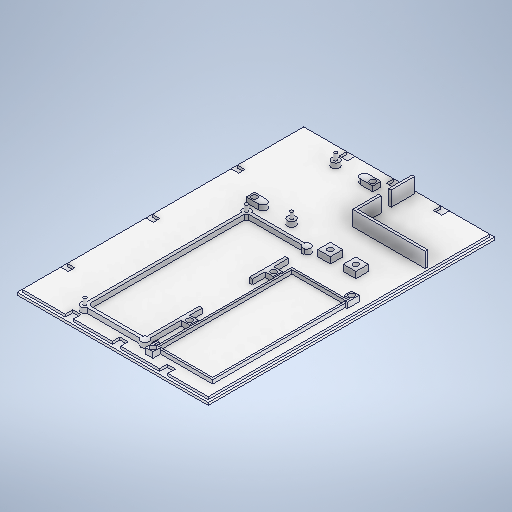
# Autodesk Inventor part: baseplate
Saved by Autodesk Inventor 2025 (Build 290162000, 162)
## iProperties
Created: 2025-05-12
Part Number: baseplate
Material: Generic
Document SubType Name: Modeling
Designer: ethan
Density: 1 g/cm^3
Appearance: PTFE
Author: ethan
Autodesk Inventor part; units mm, degrees
ref_plane "YZ Plane" through (0, 0, 0) normal (1, 0, 0) x (0, 1, 0)
ref_plane "XZ Plane" through (0, 0, 0) normal (0, 1, 0) x (-1, 0, 0)
sketch "Sketch1" plane through (0, 0, 0) normal (0, 1, 0) x (-1, 0, 0)
  line L0 (0, 0) -> (152.4, 0)
  line L1 (152.4, 0) -> (152.4, -228.6)
  line L2 (152.4, -228.6) -> (0, -228.6)
  line L3 (0, -228.6) -> (0, 0)
  dimension "d0" = 152.4
  dimension "d1" = 228.6
  constraints: 8 end point, 2 parallel, 1 horizontal, 1 perpendicular
  measures "d0" distance of L1.end L2.end
  measures "d1" distance of L0.end L1.end
extrude "BasePlate" add sketch "Sketch1" along normal blind 4
sketch "Template" plane through (0, 4, 0) normal (0, 1, 0) x (1, 0, 0)
  line L0 (0, 228.6) -> (-152.4, 228.6) construction
  line L1 (-152.4, 228.6) -> (-152.4, 0) construction
  line L2 (-152.4, 0) -> (0, 0) construction
  line L3 (0, 0) -> (0, 228.6) construction
  line L4 (-146.4, 6) -> (-146.4, 222.6) construction
  line L5 (-146.4, 222.6) -> (-6, 222.6) construction
  line L6 (-6, 222.6) -> (-6, 6) construction
  line L7 (-6, 6) -> (-146.4, 6) construction
  line L8 (-110.934, 6) -> (-110.934, 12.5) construction
  circle A0 centre (-110.934, 12.5) radius 1.25 construction
  line L9 (-110.934, 12.5) -> (-62.934, 12.5) construction
  line L10 (-62.934, 12.5) -> (-62.934, 141.5) construction
  line L11 (-62.934, 141.5) -> (-110.934, 141.5) construction
  line L12 (-110.934, 141.5) -> (-110.934, 12.5) construction
  circle A1 centre (-62.934, 12.5) radius 1.25 construction
  circle A2 centre (-110.934, 141.5) radius 1.25 construction
  circle A3 centre (-62.934, 141.5) radius 1.25 construction
  line L13 (-62.934, 12.5) -> (-6, 12.5) construction
  line L14 (-6, 12.5) -> (-9, 12.5) construction
  line L15 (-9, 12.5) -> (-55, 12.5) construction
  line L16 (-55, 12.5) -> (-55, 121.75) construction
  line L17 (-55, 121.75) -> (-9, 121.75) construction
  line L18 (-9, 121.75) -> (-9, 12.5) construction
  line L19 (-6, 222.6) -> (-63.92, 222.6) construction
  line L20 (-63.92, 222.6) -> (-63.92, 175.1) construction
  line L21 (-63.92, 175.1) -> (-6, 175.1) construction
  line L22 (-6, 175.1) -> (-6, 222.6) construction
  line L23 (-63.92, 222.6) -> (-65.92, 222.6) construction
  line L24 (-65.92, 222.6) -> (-65.92, 175.1) construction
  line L25 (-65.92, 175.1) -> (-63.92, 175.1) construction
  line L26 (-63.92, 175.1) -> (-63.92, 222.6) construction
  line L27 (-63.92, 175.1) -> (-6, 175.1) construction
  line L28 (-6, 175.1) -> (-6, 173.1) construction
  line L29 (-6, 173.1) -> (-63.92, 173.1) construction
  line L30 (-63.92, 173.1) -> (-63.92, 175.1) construction
  line L31 (-63.92, 175.1) -> (-65.92, 175.1) construction
  line L32 (-65.92, 175.1) -> (-65.92, 173.1) construction
  line L33 (-65.92, 173.1) -> (-63.92, 173.1) construction
  line L34 (-63.92, 173.1) -> (-63.92, 175.1) construction
  line L35 (-55, 121.75) -> (-55, 173.1) construction
  line L36 (-110.934, 141.5) -> (-110.934, 154.5) construction
  circle A4 centre (-110.934, 154.5) radius 1.25 construction
  line L37 (-110.934, 154.5) -> (-87.934, 154.5) construction
  line L38 (-87.934, 154.5) -> (-87.934, 212.5) construction
  line L39 (-87.934, 212.5) -> (-110.934, 212.5) construction
  line L40 (-110.934, 212.5) -> (-110.934, 154.5) construction
  circle A5 centre (-87.934, 154.5) radius 1.25 construction
  circle A6 centre (-87.934, 212.5) radius 1.25 construction
  circle A7 centre (-110.934, 212.5) radius 1.25 construction
  line L41 (-45, 142.425) -> (-55, 142.425) construction
  line L42 (-55, 142.425) -> (-55, 152.425) construction
  line L43 (-55, 152.425) -> (-45, 152.425) construction
  line L44 (-45, 152.425) -> (-45, 142.425) construction
  line L45 (-45, 142.425) -> (-55, 152.425) construction
  line L46 (-55, 142.425) -> (-45, 152.425) construction
  circle A8 centre (-50, 147.425) radius 2.25 construction
  line L47 (-50, 147.425) -> (-29.68, 147.425) construction
  line L48 (-24.68, 152.425) -> (-34.68, 152.425) construction
  line L49 (-34.68, 152.425) -> (-34.68, 142.425) construction
  line L50 (-34.68, 142.425) -> (-24.68, 142.425) construction
  line L51 (-24.68, 142.425) -> (-24.68, 152.425) construction
  line L52 (-24.68, 152.425) -> (-34.68, 142.425) construction
  line L53 (-34.68, 152.425) -> (-24.68, 142.425) construction
  dimension "d4" = 6
  dimension "d6" = 6.5
  dimension "d7" = 2.5
  dimension "d8" = 48
  dimension "d9" = 129
  dimension "d14" = 3
  dimension "d15" = 46
  dimension "d16" = 109.25
  dimension "d17" = 41.466
  dimension "d29" = 13
  dimension "d30" = 2.5
  dimension "d31" = 23
  dimension "d32" = 58
  dimension "d64" = 10
  dimension "d65" = 10
  dimension "d66" = 4.5
  dimension "d67" = 20.32
  dimension "d68" = 10
  dimension "d69" = 10
  constraints: 100 end point, 18 parallel, 12 perpendicular, 10 horizontal, 9 centre point, 8 coincident, 8 point on line, 2 midpoint, 3 other
  measures "d4" distance between parallel lines of L1 L4
  measures "d6" distance of L8.start L8.end
  measures "d7" diameter of A0
  measures "d8" distance of L11.end L10.end
  measures "d9" distance of L10.end L9.end
  measures "d14" distance of L13.end L14.end
  measures "d15" distance of L16.end L17.end
  measures "d16" distance of L15.end L16.end
  measures "d17" distance between parallel lines of L1 L12
  measures "d29" distance of L36.start L36.end
  measures "d30" diameter of A4
  measures "d31" distance of L39.end L38.end
  measures "d32" distance of L38.end L37.end
  measures "d64" distance of L42.end L43.end
  measures "d65" distance of L41.end L42.end
  measures "d66" diameter of A8
  measures "d67" distance of L47.start L47.end
  measures "d68" distance of L50.end L49.end
  measures "d69" distance of L49.end L48.end
sketch "Sketch3" plane through (0, 4, 0) normal (0, 1, 0) x (1, 0, 0)
  circle A0 centre (-110.934, 12.5) radius 1.25 construction
  circle A1 centre (-110.934, 141.5) radius 1.25 construction
  circle A2 centre (-62.934, 141.5) radius 1.25 construction
  circle A3 centre (-62.934, 12.5) radius 1.25 construction
  circle A4 centre (-110.934, 12.5) radius 3.25
  circle A5 centre (-110.934, 141.5) radius 3.25
  circle A6 centre (-62.934, 141.5) radius 3.25
  circle A7 centre (-62.934, 12.5) radius 3.25
  point P0 (0, 0)
  dimension "d37" = 2
  dimension "d38" = 2
  dimension "d39" = 2
  dimension "d40" = 2
  constraints: 4 centre point
  measures "d37" radial gap between concentric circles of A0 A4
  measures "d38" radial gap between concentric circles of A1 A5
  measures "d39" radial gap between concentric circles of A2 A6
  measures "d40" radial gap between concentric circles of A3 A7
extrude "SunFounderBase" add sketch "Sketch3" along normal blind 4
sketch "Sketch4" plane through (-110.934, 8, -12.5) normal (0, 1, 0) x (1, 0, 0)
  circle A0 centre (0, 0) radius 3.25 projected
  circle A1 centre (0, 129) radius 3.25 projected
  circle A2 centre (48, 129) radius 3.25 projected
  circle A3 centre (48, 0) radius 3.25 projected
  circle A4 centre (48, 0) radius 1.25
  circle A5 centre (0, 0) radius 1.25
  circle A6 centre (0, 129) radius 1.25
  circle A7 centre (48, 129) radius 1.25
  point P0 (110.934, -12.5)
  dimension "d43" = 2.5
  dimension "d44" = 2.5
  dimension "d45" = 2.5
  dimension "d46" = 2.5
  constraints: 4 centre point, 4 coincident
  measures "d43" diameter of A4
  measures "d44" diameter of A5
  measures "d45" diameter of A6
  measures "d46" diameter of A7
extrude "SunfounderStuds" add sketch "Sketch4" along normal blind 5 contours A5 | A6
sketch "Sketch5" plane through (0, 4, 0) normal (0, 1, 0) x (1, 0, 0)
  circle A0 centre (-110.934, 154.5) radius 1.25 construction
  circle A1 centre (-110.934, 212.5) radius 1.25 construction
  circle A2 centre (-87.934, 212.5) radius 1.25 construction
  line L0 (-87.934, 154.5) -> (-87.934, 212.5) construction
  circle A3 centre (-87.934, 154.5) radius 1.25 construction
  circle A4 centre (-87.934, 154.5) radius 3.25
  circle A5 centre (-110.934, 154.5) radius 3.25
  circle A6 centre (-110.934, 212.5) radius 3.25
  circle A7 centre (-87.934, 212.5) radius 3.25
  point P0 (0, 0)
  dimension "d49" = 2
  dimension "d50" = 2
  dimension "d51" = 2
  dimension "d52" = 2
  constraints: 4 centre point
  measures "d49" radial gap between concentric circles of A3 A4
  measures "d50" radial gap between concentric circles of A0 A5
  measures "d51" radial gap between concentric circles of A1 A6
  measures "d52" radial gap between concentric circles of A2 A7
extrude "RPiBase" add sketch "Sketch5" along normal blind 4
sketch "Sketch6" plane through (-87.934, 8, -154.5) normal (0, 1, 0) x (1, 0, 0)
  circle A0 centre (-23, 0) radius 3.25 construction
  circle A1 centre (-23, 58) radius 3.25 construction
  circle A2 centre (0, 58) radius 3.25 construction
  circle A3 centre (0, 0) radius 3.25 construction
  circle A4 centre (-23, 0) radius 1.25
  circle A5 centre (-23, 58) radius 1.25
  circle A6 centre (0, 58) radius 1.25
  circle A7 centre (0, 0) radius 1.25
  point P0 (87.934, -154.5)
  dimension "d55" = 2.5
  dimension "d56" = 2.5
  dimension "d57" = 2.5
  dimension "d58" = 2.5
  constraints: 4 centre point, 4 coincident
  measures "d55" diameter of A4
  measures "d56" diameter of A5
  measures "d57" diameter of A6
  measures "d58" diameter of A7
extrude "RPiStuds" add sketch "Sketch6" along normal blind 5 contours A5 | A7
sketch "Sketch7" plane through (0, 4, 0) normal (0, 1, 0) x (1, 0, 0)
  line L0 (-45, 142.425) -> (-55, 142.425) construction
  line L1 (-45, 152.425) -> (-45, 142.425) construction
  line L2 (-34.68, 152.425) -> (-34.68, 142.425) construction
  line L3 (-34.68, 142.425) -> (-24.68, 142.425) construction
  line L4 (-45, 142.425) -> (-55, 142.425)
  line L5 (-55, 142.425) -> (-55, 152.425)
  line L6 (-55, 152.425) -> (-45, 152.425)
  line L7 (-45, 152.425) -> (-45, 142.425)
  line L8 (-34.68, 142.425) -> (-24.68, 142.425)
  line L9 (-24.68, 142.425) -> (-24.68, 152.425)
  line L10 (-24.68, 152.425) -> (-34.68, 152.425)
  line L11 (-34.68, 152.425) -> (-34.68, 142.425)
  point P0 (0, 0)
  constraints: 16 end point, 4 parallel, 2 horizontal, 2 perpendicular, 1 point on line
extrude "VoltageConverter" add sketch "Sketch7" along normal blind 5
sketch "Sketch8" plane through (0, 9, 0) normal (0, 1, 0) x (1, 0, 0)
  line L0 (-45, 152.425) -> (-55, 152.425) projected
  line L1 (-55, 152.425) -> (-55, 142.425) projected
  line L2 (-55, 142.425) -> (-45, 142.425) projected
  line L3 (-45, 142.425) -> (-45, 152.425) projected
  line L4 (-24.68, 142.425) -> (-24.68, 152.425) projected
  line L5 (-24.68, 152.425) -> (-34.68, 152.425) projected
  line L6 (-34.68, 152.425) -> (-34.68, 142.425) projected
  line L7 (-34.68, 142.425) -> (-24.68, 142.425) projected
  circle A0 centre (-50, 147.425) radius 2.25
  circle A1 centre (-29.68, 147.425) radius 2.25
  point P0 (0, 0)
  dimension "d72" = 4.5
  dimension "d73" = 4.5
  constraints: 2 centre point
  measures "d72" diameter of A0
  measures "d73" diameter of A1
extrude "VC2" cut sketch "Sketch8" against normal blind 5 contours A0 | A1
sketch "Sketch9" plane through (0, 4, 0) normal (0, 1, 0) x (1, 0, 0)
  line L0 (-55, 12.5) -> (-55, 121.75) construction
  line L1 (-9, 12.5) -> (-55, 12.5) construction
  line L2 (-55, 12.5) -> (-9, 12.5)
  line L3 (-9, 12.5) -> (-9, 121.75)
  line L4 (-9, 121.75) -> (-55, 121.75)
  line L5 (-55, 121.75) -> (-55, 12.5)
  line L6 (-53.4, 121.75) -> (-53.4, 14.1)
  line L7 (-53.4, 14.1) -> (-9, 14.1)
  line L8 (-53.4, 120.15) -> (-10.6, 120.15)
  line L9 (-10.6, 120.15) -> (-10.6, 14.1)
  line L10 (-10.6, 14.1) -> (-53.4, 14.1)
  line L11 (-53.4, 14.1) -> (-53.4, 120.15)
  point P0 (0, 0)
  dimension "d76" = 1.6
  dimension "d77" = 1.6
  constraints: 20 end point, 4 parallel, 2 perpendicular, 1 horizontal, 4 other
  measures "d76" distance between parallel lines of L0 L6
  measures "d77" distance between parallel lines of L4 L8
extrude "12VConverter" add sketch "Sketch9" along normal blind 3 contours L5 L4 L6 L7 L3 L2 | L7 L9 L8 L6 L4 L3
sketch "Sketch10" plane through (0, 4, 0) normal (0, 1, 0) x (1, 0, 0)
  line L0 (-55, 121.75) -> (-55, 12.5) construction
  line L1 (-55, 12.5) -> (-9, 12.5) construction
  line L2 (-9, 12.5) -> (-9, 121.75) construction
  line L3 (-9, 121.75) -> (-55, 121.75) construction
  line L4 (-53.4, 120.15) -> (-10.6, 120.15) construction
  line L5 (-10.6, 120.15) -> (-10.6, 14.1) construction
  line L6 (-10.6, 14.1) -> (-53.4, 14.1) construction
  line L7 (-53.4, 14.1) -> (-53.4, 120.15) construction
  line L8 (-56.6, 10.9) -> (-56.6, 123.35) construction
  line L9 (-56.6, 123.35) -> (-7.4, 123.35) construction
  line L10 (-7.4, 123.35) -> (-7.4, 10.9) construction
  line L11 (-7.4, 10.9) -> (-56.6, 10.9) construction
  line L12 (-56.6, 10.9) -> (-51.6, 10.9) construction
  line L13 (-51.6, 10.9) -> (-51.6, 15.9) construction
  line L14 (-51.6, 15.9) -> (-56.6, 15.9) construction
  line L15 (-56.6, 15.9) -> (-56.6, 10.9) construction
  line L16 (-51.6, 10.9) -> (-51.6, 12.5)
  line L17 (-55, 12.5) -> (-51.6, 12.5)
  line L18 (-55, 12.5) -> (-55, 15.9)
  line L19 (-55, 15.9) -> (-56.6, 15.9)
  line L20 (-56.6, 15.9) -> (-56.6, 10.9)
  line L21 (-56.6, 10.9) -> (-51.6, 10.9)
  line L22 (-7.4, 123.35) -> (-12.4, 123.35)
  line L23 (-12.4, 123.35) -> (-12.4, 118.35)
  line L24 (-12.4, 118.35) -> (-7.4, 118.35)
  line L25 (-7.4, 118.35) -> (-7.4, 123.35)
  line L26 (-9, 121.75) -> (-55, 121.75) projected
  line L27 (-12.4, 121.75) -> (-9, 121.75)
  line L28 (-9, 121.75) -> (-9, 118.35)
  point P0 (0, 0)
  dimension "d80" = 1.6
  dimension "d81" = 5
  dimension "d82" = 5
  dimension "d83" = 5
  dimension "d84" = 5
  constraints: 40 end point, 8 point on line, 4 parallel, 4 perpendicular, 3 collinear, 2 horizontal, 3 other
  measures "d80" distance between parallel lines of L0 L8
  measures "d81" distance of L14.end L13.end
  measures "d82" distance of L13.end L12.end
  measures "d83" distance of L24.end L23.end
  measures "d84" distance of L23.end L22.end
extrude "12V2" add sketch "Sketch10" along normal blind 4.5 contours L21 L20 L19 L18 L17 L16 | L25 L24 L28 L26 L23 L22
sketch "Sketch11" plane through (0, 4, 0) normal (0, 1, 0) x (1, 0, 0)
  line L0 (0, 0) -> (0, 228.6) projected
  line L1 (-59.92, 226.6) -> (-61.92, 226.6)
  line L2 (-61.92, 226.6) -> (-61.92, 177.1)
  line L3 (-61.92, 177.1) -> (-2, 177.1)
  line L4 (-2, 177.1) -> (-2, 179.1)
  line L5 (0, 228.6) -> (-152.4, 228.6) projected
  line L6 (-59.92, 179.1) -> (-59.92, 224.6)
  line L7 (-4, 179.1) -> (-59.92, 179.1)
  line L8 (-59.92, 224.6) -> (-59.92, 226.6)
  line L9 (-4, 179.1) -> (-2, 179.1)
  line L10 (-2, 177.1) -> (-4, 177.1)
  line L11 (-4, 177.1) -> (-4, 179.1)
  line L12 (-4, 179.1) -> (-2, 179.1)
  line L13 (-2, 179.1) -> (-2, 177.1)
  line L14 (-61.92, 226.6) -> (-59.92, 226.6)
  line L15 (-59.92, 226.6) -> (-59.92, 224.6)
  line L16 (-59.92, 224.6) -> (-61.92, 224.6)
  line L17 (-61.92, 224.6) -> (-61.92, 226.6)
  dimension "d114" = 59.92
  dimension "d115" = 49.5
  dimension "d116" = 2
  dimension "d117" = 2
  dimension "d118" = 2
  dimension "d179" = 2
  dimension "d180" = 2
  constraints: 32 end point, 6 parallel, 4 perpendicular, 3 horizontal, 1 vertical
  measures "d114" distance of L3.end L2.end
  measures "d115" distance of L2.end L1.end
  measures "d116" distance between parallel lines of L5 L1
  measures "d117" distance between parallel lines of L0 L4
  measures "d118" distance between parallel lines of L2 L6
  measures "d179" distance of L7.start L12.end
  measures "d180" distance of L14.end L6.end
extrude "PoEBlock" add sketch "Sketch11" along normal blind 12 contours L6 L7 L11 L3 L2 L16
sketch "Sketch14" plane through (0, 4, 0) normal (0, 1, 0) x (1, 0, 0)
  circle A0 centre (-110.934, 12.5) radius 1.25 projected
  circle A1 centre (-110.934, 141.5) radius 1.25 projected
  line L0 (-62.934, 142.75) -> (-110.934, 142.75)
  circle A2 centre (-62.934, 141.5) radius 1.25 projected
  line L1 (-112.184, 141.5) -> (-112.184, 12.5)
  line L2 (-110.934, 11.25) -> (-62.934, 11.25)
  line L3 (-61.684, 12.5) -> (-61.684, 141.5)
  line L4 (-61.684, 142.75) -> (-64.184, 142.75) construction
  line L5 (-64.184, 142.75) -> (-64.184, 140.25) construction
  line L6 (-64.184, 140.25) -> (-61.684, 140.25) construction
  line L7 (-61.684, 140.25) -> (-61.684, 142.75) construction
  line L8 (-64.184, 140.25) -> (-110.934, 140.25) construction
  line L9 (-64.184, 141.5) -> (-64.184, 12.5)
  line L10 (-62.934, 13.75) -> (-110.934, 13.75)
  line L11 (-109.684, 12.5) -> (-109.684, 141.5)
  line L12 (-110.934, 140.25) -> (-62.934, 140.25)
  line L13 (-110.934, 11.25) -> (-61.684, 11.25)
  line L14 (-61.684, 11.25) -> (-61.684, 13.75)
  line L15 (-61.684, 13.75) -> (-110.934, 13.75)
  line L16 (-110.934, 13.75) -> (-110.934, 11.25)
  line L17 (-61.684, 11.25) -> (-64.184, 11.25)
  line L18 (-64.184, 11.25) -> (-64.184, 142.75)
  line L19 (-64.184, 142.75) -> (-61.684, 142.75)
  line L20 (-61.684, 142.75) -> (-61.684, 11.25)
  line L21 (-112.6766, 140.25) -> (-61.684, 140.25)
  line L22 (-61.684, 140.25) -> (-61.684, 142.75)
  line L23 (-61.684, 142.75) -> (-112.6766, 142.75)
  line L24 (-112.6766, 142.75) -> (-112.6766, 140.25)
  point P0 (0, 0)
  point P1 (-64.184, 13.75)
  point P2 (-109.684, 140.25)
  point P3 (-109.684, 13.75)
  point P4 (-112.184, 140.25)
  point P5 (-64.184, 12.5)
  constraints: 50 end point, 9 point on circle, 8 parallel, 7 tangent, 6 horizontal, 4 perpendicular, 3 point on line, 2 midpoint
extrude "SunfounderSupport" add sketch "Sketch14" along normal blind 4 contours L11 L10 L9 L18 L2 A0 | A0 L10 L11 | A0 L1 L21 L12 L11 L10 | L9 L12 L21 L3 L15 L10 | L12 A1 L11 | L11 A1 L0 L18 L9 L12 | L21 L24 L23 A1 L1 | L1 A1 L21 | L9 A2 L12 | A1 | L18 L0 A2 | A2 | A2 L3 L21 | L19 L20 A2
sketch "Sketch15" plane through (0, 8, 0) normal (0, 1, 0) x (1, 0, 0)
  arc A0 (-107.934, 142.75) -> (-112.184, 138.5) centre (-110.934, 141.5) ccw projected
  line L0 (-112.184, 138.5) -> (-112.184, 15.5) projected
  arc A1 (-112.184, 15.5) -> (-107.934, 11.25) centre (-110.934, 12.5) ccw projected
  arc A2 (-65.934, 11.25) -> (-61.684, 15.5) centre (-62.934, 12.5) ccw projected
  arc A3 (-61.684, 138.5) -> (-65.934, 142.75) centre (-62.934, 141.5) ccw projected
  circle A4 centre (-110.934, 12.5) radius 1.25 projected
  line L1 (-109.684, 15.5) -> (-109.684, 138.5) projected
  circle A5 centre (-110.934, 141.5) radius 1.25 projected
  line L2 (-61.684, 138.5) -> (-61.684, 15.5) projected
  line L3 (-64.184, 138.5) -> (-61.684, 138.5)
  line L4 (-61.684, 138.5) -> (-61.684, 125.5)
  line L5 (-61.684, 125.5) -> (-64.184, 125.5)
  line L6 (-64.184, 125.5) -> (-64.184, 138.5)
  line L7 (-66.684, 57) -> (-66.684, 97)
  line L8 (-66.684, 97) -> (-61.684, 97)
  line L9 (-61.684, 97) -> (-61.684, 57)
  line L10 (-61.684, 57) -> (-66.684, 57)
  line L11 (-66.684, 57) -> (-61.684, 97) construction
  line L12 (-66.684, 97) -> (-61.684, 57) construction
  arc A6 (-107.934, 13.75) -> (-109.684, 15.5) centre (-110.934, 12.5) ccw projected
  arc A7 (-109.684, 138.5) -> (-107.934, 140.25) centre (-110.934, 141.5) ccw projected
  line L13 (-107.934, 140.25) -> (-65.934, 140.25) projected
  arc A8 (-65.934, 140.25) -> (-64.184, 138.5) centre (-62.934, 141.5) ccw projected
  line L14 (-64.184, 138.5) -> (-64.184, 15.5) projected
  arc A9 (-64.184, 15.5) -> (-65.934, 13.75) centre (-62.934, 12.5) ccw projected
  line L15 (-65.934, 13.75) -> (-107.934, 13.75) projected
  line L16 (-107.934, 11.25) -> (-65.934, 11.25) projected
  line L17 (-61.684, 15.5) -> (-61.684, 138.5) projected
  line L18 (-65.934, 142.75) -> (-107.934, 142.75) projected
  point P0 (0, 0)
  point P1 (-64.184, 77)
  dimension "d98" = 13
  dimension "d99" = 40
  constraints: 20 end point, 4 parallel, 2 midpoint, 2 perpendicular, 1 horizontal, 1 point on line
  measures "d98" distance of L3.end L4.end
  measures "d99" distance of L7.start L7.end
extrude "SS2" cut sketch "Sketch15" against normal up to surface (4 mm away) contours L2 L5 L6 L3 | L2 L10 L14 L8 | L14 L10 L7 L8
sketch "Sketch16" plane through (0, 4, 0) normal (0, 1, 0) x (1, 0, 0)
  line L0 (-55, 15.9) -> (-56.6, 15.9) projected
  line L1 (-56.6, 15.9) -> (-56.6, 10.9) projected
  line L2 (-56.6, 10.9) -> (-51.6, 10.9) projected
  line L3 (-51.6, 10.9) -> (-51.6, 12.5) projected
  line L4 (-51.6, 12.5) -> (-55, 12.5) projected
  line L5 (-55, 12.5) -> (-55, 15.9) projected
  line L6 (-6, 6) -> (-146.4, 6) construction
  line L7 (-51.6, 10.9) -> (-56.6, 10.9)
  line L8 (-56.6, 10.9) -> (-56.6, 6.5)
  line L9 (-56.6, 6.5) -> (-51.6, 6.5)
  line L10 (-51.6, 6.5) -> (-51.6, 10.9)
  line L11 (-9, 12.5) -> (-51.6, 12.5) projected
  line L12 (-51.6, 6.5) -> (-50.6, 6.5)
  line L13 (-50.6, 6.5) -> (-50.6, 12.5)
  line L14 (-50.6, 12.5) -> (-51.6, 12.5)
  line L15 (-51.6, 12.5) -> (-51.6, 6.5)
  line L16 (-7.4, 123.35) -> (-12.4, 123.35) projected
  line L17 (-7.4, 123.35) -> (-7.4, 118.35) projected
  line L18 (-7.4, 123.35) -> (-13.4, 123.35)
  line L19 (-13.4, 123.35) -> (-13.4, 127.75)
  line L20 (-13.4, 127.75) -> (-7.4, 127.75)
  line L21 (-7.4, 127.75) -> (-7.4, 123.35)
  line L22 (-12.4, 121.75) -> (-12.4, 123.35) projected
  line L23 (-13.4, 123.35) -> (-12.4, 123.35)
  line L24 (-12.4, 123.35) -> (-12.4, 121.75)
  line L25 (-12.4, 121.75) -> (-13.4, 121.75)
  line L26 (-13.4, 121.75) -> (-13.4, 123.35)
  point P0 (0, 0)
  dimension "d102" = 4.4
  dimension "d103" = 1
  dimension "d104" = 6
  dimension "d105" = 4.4
  constraints: 32 end point, 8 parallel, 4 horizontal, 4 perpendicular, 1 point on line
  measures "d102" distance of L8.end L7.end
  measures "d103" distance of L14.end L13.end
  measures "d104" distance of L19.end L20.end
  measures "d105" distance of L18.end L19.end
extrude "Latch12V" add sketch "Sketch16" along normal blind 4.5 contours L2 L10 L9 L8 | L11 L13 L12 L10 L3 | L16 L18 L19 L20 L21 | L22 L25 L26 L18
sketch "Sketch17" plane through (0, 8.5, 0) normal (0, 1, 0) x (1, 0, 0)
  line L0 (-55, 15.9) -> (-56.6, 15.9) projected
  line L1 (-56.6, 15.9) -> (-56.6, 6.5) projected
  line L2 (-56.6, 6.5) -> (-50.6, 6.5) projected
  line L3 (-50.6, 6.5) -> (-50.6, 12.5) projected
  line L4 (-50.6, 12.5) -> (-55, 12.5) projected
  line L5 (-55, 12.5) -> (-55, 15.9) projected
  circle A0 centre (-53.6, 9.5) radius 2.25
  line L6 (-13.4, 121.75) -> (-9, 121.75) projected
  line L7 (-9, 121.75) -> (-9, 118.35) projected
  line L8 (-9, 118.35) -> (-7.4, 118.35) projected
  line L9 (-7.4, 118.35) -> (-7.4, 127.75) projected
  line L10 (-7.4, 127.75) -> (-13.4, 127.75) projected
  line L11 (-13.4, 127.75) -> (-13.4, 121.75) projected
  circle A1 centre (-10.4, 124.75) radius 2.25
  point P0 (0, 0)
  dimension "d108" = 4.5
  dimension "d109" = 4.5
  constraints: 2 centre point
  measures "d108" diameter of A0
  measures "d109" diameter of A1
extrude "L12V2" cut sketch "Sketch17" against normal blind 5 contours A0 | A1
sketch "Sketch18" plane through (0, 4, 0) normal (0, 1, 0) x (1, 0, 0)
  line L0 (-56.6, 6.5) -> (-56.6, 15.9) construction
  line L1 (-56.6, 15.9) -> (-55, 15.9) construction
  line L2 (-55, 15.9) -> (-55, 121.75) construction
  line L3 (-55, 121.75) -> (-13.4, 121.75) construction
  line L4 (-13.4, 121.75) -> (-13.4, 127.75) construction
  line L5 (-13.4, 127.75) -> (-7.4, 127.75) construction
  line L6 (-7.4, 127.75) -> (-7.4, 118.35) construction
  line L7 (-7.4, 118.35) -> (-9, 118.35) construction
  line L8 (-9, 118.35) -> (-9, 12.5) construction
  line L9 (-9, 12.5) -> (-50.6, 12.5) construction
  line L10 (-50.6, 12.5) -> (-50.6, 6.5) construction
  line L11 (-50.6, 6.5) -> (-56.6, 6.5) construction
  arc A0 (-65.934, 140.25) -> (-64.184, 138.5) centre (-62.934, 141.5) ccw construction
  arc A1 (-109.684, 138.5) -> (-107.934, 140.25) centre (-110.934, 141.5) ccw construction
  line L12 (-109.684, 138.5) -> (-109.684, 15.5) construction
  arc A2 (-107.934, 13.75) -> (-109.684, 15.5) centre (-110.934, 12.5) ccw construction
  arc A3 (-64.184, 15.5) -> (-65.934, 13.75) centre (-62.934, 12.5) ccw construction
  line L13 (-112.184, 15.5) -> (-112.184, 138.5) construction
  line L14 (-64.184, 138.5) -> (-61.684, 138.5) construction
  line L15 (-59.92, 179.1) -> (-4, 179.1) construction
  line L16 (-4, 177.1) -> (-61.92, 177.1) construction
  line L17 (-61.92, 177.1) -> (-61.92, 224.6) construction
  line L18 (-59.92, 224.6) -> (-59.92, 179.1) construction
  line L19 (-24.68, 142.425) -> (-34.68, 142.425) construction
  line L20 (-34.68, 142.425) -> (-34.68, 152.425) construction
  line L21 (-34.68, 152.425) -> (-24.68, 152.425) construction
  line L22 (-24.68, 152.425) -> (-24.68, 142.425) construction
  line L23 (-45, 152.425) -> (-45, 142.425) construction
  line L24 (-45, 142.425) -> (-55, 142.425) construction
  line L25 (-55, 142.425) -> (-55, 152.425) construction
  line L26 (-55, 152.425) -> (-45, 152.425) construction
  circle A4 centre (-110.934, 212.5) radius 3.25 construction
  circle A5 centre (-110.934, 154.5) radius 3.25 construction
  circle A6 centre (-87.934, 154.5) radius 3.25 construction
  circle A7 centre (-87.934, 212.5) radius 3.25 construction
  line L27 (0, 228.6) -> (-152.4, 228.6) construction
  line L28 (-152.4, 228.6) -> (-152.4, 0) construction
  line L29 (-152.4, 0) -> (0, 0) construction
  line L30 (0, 0) -> (0, 228.6) construction
  circle A8 centre (-110.934, 154.5) radius 3.25 construction
  line L31 (-110.934, 151.25) -> (-120.934, 151.25) construction
  line L32 (-120.934, 151.25) -> (-120.934, 157.75) construction
  line L33 (-120.934, 157.75) -> (-110.934, 157.75) construction
  line L34 (-110.934, 157.75) -> (-110.934, 151.25) construction
  line L35 (-87.934, 209.25) -> (-77.934, 209.25) construction
  line L36 (-77.934, 209.25) -> (-77.934, 215.75) construction
  line L37 (-77.934, 215.75) -> (-87.934, 215.75) construction
  line L38 (-87.934, 215.75) -> (-87.934, 209.25) construction
  line L39 (-110.934, 151.25) -> (-120.934, 151.25) construction
  line L40 (-120.934, 151.25) -> (-120.934, 157.75) construction
  line L41 (-120.934, 157.75) -> (-110.934, 157.75) construction
  line L42 (-110.934, 157.75) -> (-110.934, 151.25) construction
  line L43 (-120.934, 151.25) -> (-110.934, 151.25)
  line L44 (-110.934, 151.25) -> (-110.934, 157.75)
  line L45 (-110.934, 157.75) -> (-120.934, 157.75)
  line L46 (-120.934, 157.75) -> (-120.934, 151.25)
  line L47 (-87.934, 209.25) -> (-77.934, 209.25)
  line L48 (-77.934, 209.25) -> (-77.934, 215.75)
  line L49 (-77.934, 215.75) -> (-87.934, 215.75)
  line L50 (-87.934, 215.75) -> (-87.934, 209.25)
  line L51 (-120.934, 151.25) -> (-114.184, 151.25) construction
  line L52 (-114.184, 151.25) -> (-114.184, 157.75) construction
  line L53 (-114.184, 157.75) -> (-120.934, 157.75) construction
  line L54 (-120.934, 157.75) -> (-120.934, 151.25) construction
  circle A9 centre (-117.559, 154.5) radius 2.25 construction
  circle A10 centre (-117.559, 154.5) radius 2.25
  line L55 (-84.684, 215.75) -> (-77.934, 215.75) construction
  line L56 (-77.934, 215.75) -> (-77.934, 209.25) construction
  line L57 (-77.934, 209.25) -> (-84.684, 209.25) construction
  line L58 (-84.684, 209.25) -> (-84.684, 215.75) construction
  circle A11 centre (-81.309, 212.5) radius 2.25 construction
  circle A12 centre (-81.309, 212.5) radius 2.25
  line L59 (-65.934, 140.25) -> (-107.934, 140.25) projected
  line L60 (-107.934, 13.75) -> (-65.934, 13.75) projected
  line L61 (-64.184, 15.5) -> (-64.184, 57) projected
  line L62 (-61.684, 57) -> (-64.184, 57) projected
  line L63 (-61.684, 57) -> (-61.684, 15.5) projected
  arc A13 (-65.934, 11.25) -> (-61.684, 15.5) centre (-62.934, 12.5) ccw projected
  line L64 (-65.934, 11.25) -> (-107.934, 11.25) projected
  arc A14 (-112.184, 15.5) -> (-107.934, 11.25) centre (-110.934, 12.5) ccw projected
  arc A15 (-107.934, 142.75) -> (-112.184, 138.5) centre (-110.934, 141.5) ccw projected
  line L65 (-107.934, 142.75) -> (-65.934, 142.75) projected
  arc A16 (-61.684, 138.5) -> (-65.934, 142.75) centre (-62.934, 141.5) ccw projected
  line L66 (-4, 179.1) -> (-4, 177.1) projected
  line L67 (-61.92, 224.6) -> (-59.92, 224.6) projected
  dimension "d119" = 10
  dimension "d120" = 10
  dimension "d121" = 4.5
  dimension "d122" = 4.5
  constraints: 56 end point, 14 parallel, 7 horizontal, 7 perpendicular, 4 centre point, 2 coincident, 2 concentric, 2 point on line, 2 vertical alignment, 2 other
  measures "d119" distance of L32.end L33.end
  measures "d120" distance of L37.end L36.end
  measures "d121" diameter of A9
  measures "d122" diameter of A11
extrude "LatchRpi" add sketch "Sketch18" along normal blind 4
sketch "Sketch19" plane through (-117.559, 4, -154.5) normal (0, 1, 0) x (1, 0, 0)
  circle A0 centre (0, 0) radius 2.25 projected
  circle A1 centre (36.25, 58) radius 2.25 projected
  point P0 (117.559, -154.5)
extrude "LP2" cut sketch "Sketch19" against normal blind 1
sketch "Sketch20" plane through (0, 4, 0) normal (0, 1, 0) x (1, 0, 0)
  arc A0 (-64.184, 15.5) -> (-65.934, 13.75) centre (-62.934, 12.5) ccw projected
  arc A1 (-65.934, 140.25) -> (-64.184, 138.5) centre (-62.934, 141.5) ccw projected
  line L0 (-62.934, 12.5) -> (-62.934, 141.5) construction
  line L1 (-62.934, 77) -> (-62.934, 47) construction
  line L2 (-62.934, 47) -> (-62.934, 107) construction
  line L3 (-55, 121.75) -> (-55, 15.9) construction
  line L4 (-62.934, 47) -> (-55, 47) construction
  line L5 (-55, 47) -> (-55, 40) construction
  line L6 (-55, 40) -> (-62.934, 40) construction
  line L7 (-62.934, 40) -> (-62.934, 47) construction
  line L8 (-64.184, 15.5) -> (-64.184, 57) construction
  line L9 (-55, 40) -> (-64.184, 40) construction
  line L10 (-64.184, 40) -> (-64.184, 47) construction
  line L11 (-64.184, 47) -> (-55, 47) construction
  line L12 (-55, 47) -> (-55, 40) construction
  line L13 (-62.934, 107) -> (-55, 107) construction
  line L14 (-55, 107) -> (-55, 114) construction
  line L15 (-55, 114) -> (-62.934, 114) construction
  line L16 (-62.934, 114) -> (-62.934, 107) construction
  line L17 (-55, 114) -> (-62.934, 114)
  line L18 (-62.934, 114) -> (-62.934, 107)
  line L19 (-62.934, 107) -> (-55, 107)
  line L20 (-55, 107) -> (-55, 114)
  line L21 (-62.934, 47) -> (-55, 47)
  line L22 (-55, 47) -> (-55, 40)
  line L23 (-55, 40) -> (-62.934, 40)
  line L24 (-62.934, 40) -> (-62.934, 47)
  point P0 (0, 0)
  dimension "d127" = 30
  dimension "d128" = 60
  dimension "d129" = 7
  dimension "d130" = 7
  constraints: 46 end point, 10 parallel, 5 horizontal, 5 perpendicular, 5 point on line, 1 midpoint, 1 vertical
  measures "d127" distance of L1.start L1.end
  measures "d128" distance of L1.end L2.end
  measures "d129" distance of L4.end L5.end
  measures "d130" distance of L14.end L13.end
extrude "LatchSunF" add sketch "Sketch20" along normal blind 4
sketch "Sketch21" plane through (0, 8, 0) normal (0, 1, 0) x (1, 0, 0)
  line L0 (-61.684, 47) -> (-61.684, 57) construction
  line L1 (-61.684, 57) -> (-64.184, 57) construction
  line L2 (-64.184, 57) -> (-64.184, 15.5) construction
  arc A0 (-64.184, 15.5) -> (-65.934, 13.75) centre (-62.934, 12.5) ccw construction
  line L3 (-65.934, 13.75) -> (-107.934, 13.75) construction
  arc A1 (-107.934, 13.75) -> (-109.684, 15.5) centre (-110.934, 12.5) ccw construction
  line L4 (-109.684, 15.5) -> (-109.684, 138.5) construction
  arc A2 (-109.684, 138.5) -> (-107.934, 140.25) centre (-110.934, 141.5) ccw construction
  line L5 (-107.934, 140.25) -> (-65.934, 140.25) construction
  arc A3 (-65.934, 140.25) -> (-64.184, 138.5) centre (-62.934, 141.5) ccw construction
  line L6 (-64.184, 138.5) -> (-61.684, 138.5) construction
  arc A4 (-61.684, 138.5) -> (-65.934, 142.75) centre (-62.934, 141.5) ccw construction
  line L7 (-65.934, 142.75) -> (-107.934, 142.75) construction
  arc A5 (-107.934, 142.75) -> (-112.184, 138.5) centre (-110.934, 141.5) ccw construction
  line L8 (-112.184, 138.5) -> (-112.184, 15.5) construction
  arc A6 (-112.184, 15.5) -> (-107.934, 11.25) centre (-110.934, 12.5) ccw construction
  line L9 (-107.934, 11.25) -> (-65.934, 11.25) construction
  arc A7 (-65.934, 11.25) -> (-61.684, 15.5) centre (-62.934, 12.5) ccw construction
  line L10 (-61.684, 15.5) -> (-61.684, 40) construction
  line L11 (-61.684, 40) -> (-55, 40) construction
  line L12 (-55, 40) -> (-55, 47) construction
  line L13 (-55, 47) -> (-61.684, 47) construction
  circle A8 centre (-110.934, 141.5) radius 1.25 construction
  circle A9 centre (-110.934, 12.5) radius 1.25 construction
  line L14 (-61.684, 114) -> (-61.684, 125.5) construction
  line L15 (-61.684, 125.5) -> (-64.184, 125.5) construction
  line L16 (-64.184, 125.5) -> (-64.184, 97) construction
  line L17 (-64.184, 97) -> (-61.684, 97) construction
  line L18 (-61.684, 97) -> (-61.684, 107) construction
  line L19 (-61.684, 107) -> (-55, 107) construction
  line L20 (-55, 107) -> (-55, 114) construction
  line L21 (-55, 114) -> (-61.684, 114) construction
  circle A10 centre (-58.342, 43.5) radius 2.25 construction
  circle A11 centre (-58.342, 43.5) radius 2.25
  circle A12 centre (-58.342, 110.5) radius 2.25
  point P0 (0, 0)
  dimension "d133" = 4.5
  dimension "d134" = 4.5
  constraints: 3 centre point, 1 coincident, 1 concentric
  measures "d133" diameter of A10
  measures "d134" diameter of A12
extrude "LatchSunF2" cut sketch "Sketch21" against normal blind 5
sketch "Sketch22" plane through (0, 16, 0) normal (0, 1, 0) x (1, 0, 0)
  line L0 (-59.92, 179.1) -> (-59.92, 224.6) projected
  line L1 (-61.92, 224.6) -> (-61.92, 177.1) projected
  line L2 (-61.92, 177.1) -> (-4, 177.1) projected
  line L3 (-4, 179.1) -> (-59.92, 179.1) projected
  line L4 (-59.92, 201.85) -> (-61.92, 201.85) construction
  line L5 (-61.92, 197.85) -> (-59.92, 197.85) construction
  line L6 (-59.92, 197.85) -> (-59.92, 205.85) construction
  line L7 (-59.92, 205.85) -> (-61.92, 205.85) construction
  line L8 (-61.92, 205.85) -> (-61.92, 197.85) construction
  line L9 (-61.92, 197.85) -> (-59.92, 205.85) construction
  line L10 (-59.92, 197.85) -> (-61.92, 205.85) construction
  line L11 (-59.92, 197.85) -> (-61.92, 197.85)
  line L12 (-61.92, 197.85) -> (-61.92, 205.85)
  line L13 (-61.92, 205.85) -> (-59.92, 205.85)
  line L14 (-59.92, 205.85) -> (-59.92, 197.85)
  line L15 (-4, 177.1) -> (-4, 179.1) projected
  line L16 (-59.92, 224.6) -> (-61.92, 224.6) projected
  point P0 (0, 0)
  point P1 (-60.92, 201.85)
  point P2 (-61.92, 205.85)
  point P3 (-61.92, 197.85)
  dimension "d137" = 8
  constraints: 22 end point, 4 midpoint, 4 parallel, 3 perpendicular, 2 horizontal, 2 point on line
  measures "d137" distance of L6.end L5.end
extrude "PoERemove" cut sketch "Sketch22" against normal up to surface (12 mm away) contours L11 L1 L13 L0
sketch "Sketch23" plane through (0, 4, 0) normal (0, 1, 0) x (1, 0, 0)
  line L0 (-61.92, 205.85) -> (-61.92, 224.6) construction
  line L1 (-59.92, 224.6) -> (-59.92, 205.85) construction
  line L2 (-61.92, 205.85) -> (-59.92, 205.85) construction
  line L3 (-61.684, 114) -> (-55, 114) construction
  line L4 (-55, 114) -> (-55, 121.75) construction
  line L5 (-55, 121.75) -> (-13.4, 121.75) construction
  line L6 (-13.4, 121.75) -> (-13.4, 127.75) construction
  line L7 (-13.4, 127.75) -> (-7.4, 127.75) construction
  line L8 (-7.4, 127.75) -> (-7.4, 118.35) construction
  line L9 (-7.4, 118.35) -> (-9, 118.35) construction
  line L10 (-9, 118.35) -> (-9, 12.5) construction
  line L11 (-9, 12.5) -> (-50.6, 12.5) construction
  line L12 (-50.6, 12.5) -> (-50.6, 6.5) construction
  line L13 (-50.6, 6.5) -> (-56.6, 6.5) construction
  line L14 (-56.6, 6.5) -> (-56.6, 15.9) construction
  line L15 (-56.6, 15.9) -> (-55, 15.9) construction
  line L16 (-55, 15.9) -> (-55, 40) construction
  line L17 (-55, 40) -> (-61.684, 40) construction
  line L18 (-61.684, 40) -> (-61.684, 15.5) construction
  arc A0 (-65.934, 11.25) -> (-61.684, 15.5) centre (-62.934, 12.5) ccw construction
  line L19 (-65.934, 11.25) -> (-107.934, 11.25) construction
  arc A1 (-112.184, 15.5) -> (-107.934, 11.25) centre (-110.934, 12.5) ccw construction
  line L20 (-112.184, 15.5) -> (-112.184, 138.5) construction
  arc A2 (-107.934, 142.75) -> (-112.184, 138.5) centre (-110.934, 141.5) ccw construction
  line L21 (-107.934, 142.75) -> (-65.934, 142.75) construction
  arc A3 (-61.684, 138.5) -> (-65.934, 142.75) centre (-62.934, 141.5) ccw construction
  line L22 (-64.184, 138.5) -> (-61.684, 138.5) construction
  arc A4 (-65.934, 140.25) -> (-64.184, 138.5) centre (-62.934, 141.5) ccw construction
  line L23 (-65.934, 140.25) -> (-107.934, 140.25) construction
  arc A5 (-109.684, 138.5) -> (-107.934, 140.25) centre (-110.934, 141.5) ccw construction
  line L24 (-109.684, 138.5) -> (-109.684, 15.5) construction
  arc A6 (-107.934, 13.75) -> (-109.684, 15.5) centre (-110.934, 12.5) ccw construction
  line L25 (-107.934, 13.75) -> (-65.934, 13.75) construction
  arc A7 (-64.184, 15.5) -> (-65.934, 13.75) centre (-62.934, 12.5) ccw construction
  line L26 (-64.184, 15.5) -> (-64.184, 57) construction
  line L27 (-61.684, 57) -> (-64.184, 57) construction
  line L28 (-61.684, 57) -> (-61.684, 47) construction
  line L29 (-61.684, 47) -> (-55, 47) construction
  line L30 (-55, 47) -> (-55, 107) construction
  line L31 (-55, 107) -> (-61.684, 107) construction
  line L32 (-61.684, 107) -> (-61.684, 97) construction
  line L33 (-64.184, 97) -> (-61.684, 97) construction
  line L34 (-64.184, 97) -> (-64.184, 125.5) construction
  line L35 (-61.684, 125.5) -> (-64.184, 125.5) construction
  line L36 (-61.684, 125.5) -> (-61.684, 114) construction
  line L37 (-77.934, 209.25) -> (-87.934, 209.25) construction
  arc A8 (-87.934, 215.75) -> (-87.934, 209.25) centre (-87.934, 212.5) ccw construction
  line L38 (-87.934, 215.75) -> (-77.934, 215.75) construction
  line L39 (-77.934, 215.75) -> (-77.934, 209.25) construction
  line L40 (-120.934, 157.75) -> (-110.934, 157.75) construction
  arc A9 (-110.934, 151.25) -> (-110.934, 157.75) centre (-110.934, 154.5) ccw construction
  line L41 (-110.934, 151.25) -> (-120.934, 151.25) construction
  line L42 (-120.934, 151.25) -> (-120.934, 157.75) construction
  line L43 (-59.92, 197.85) -> (-61.92, 197.85) construction
  line L44 (-59.92, 197.85) -> (-59.92, 179.1) construction
  line L45 (-59.92, 179.1) -> (-4, 179.1) construction
  line L46 (-4, 177.1) -> (-61.92, 177.1) construction
  line L47 (-61.92, 177.1) -> (-61.92, 197.85) construction
  line L48 (-24.68, 142.425) -> (-34.68, 142.425) construction
  line L49 (-34.68, 142.425) -> (-34.68, 152.425) construction
  line L50 (-34.68, 152.425) -> (-24.68, 152.425) construction
  line L51 (-24.68, 152.425) -> (-24.68, 142.425) construction
  line L52 (-45, 152.425) -> (-45, 142.425) construction
  line L53 (-45, 142.425) -> (-55, 142.425) construction
  line L54 (-55, 142.425) -> (-55, 152.425) construction
  line L55 (-55, 152.425) -> (-45, 152.425) construction
  circle A10 centre (-110.934, 212.5) radius 3.25 construction
  circle A11 centre (-87.934, 154.5) radius 3.25 construction
  line L56 (0, 228.6) -> (-152.4, 228.6) construction
  line L57 (-152.4, 228.6) -> (-152.4, 0) construction
  line L58 (-152.4, 0) -> (0, 0) construction
  line L59 (0, 0) -> (0, 228.6) construction
  line L60 (-150.4, 2) -> (-150.4, 226.6) construction
  line L61 (-150.4, 226.6) -> (-2, 226.6) construction
  line L62 (-2, 226.6) -> (-2, 2) construction
  line L63 (-2, 2) -> (-150.4, 2) construction
  line L64 (-152.4, 228.6) -> (-152.4, 0) projected
  line L65 (-152.4, 0) -> (0, 0)
  line L66 (0, 0) -> (0, 228.6)
  line L67 (0, 228.6) -> (-152.4, 228.6)
  line L68 (-152.4, 228.6) -> (-152.4, 0)
  line L69 (-2, 226.6) -> (-150.4, 226.6)
  line L70 (-150.4, 226.6) -> (-150.4, 2)
  line L71 (-150.4, 2) -> (-2, 2)
  line L72 (-2, 2) -> (-2, 226.6)
  line L73 (-4, 179.1) -> (-4, 177.1) projected
  line L74 (-61.92, 224.6) -> (-59.92, 224.6) projected
  dimension "d140" = 2
  constraints: 24 end point, 4 parallel, 2 horizontal, 2 perpendicular, 3 other
  measures "d140" distance between parallel lines of L57 L60
extrude "EdgeCut" cut sketch "Sketch23" against normal blind 2
sketch "Sketch24" plane through (0, 4, 0) normal (0, 1, 0) x (1, 0, 0)
  line L0 (-152.4, 0) -> (-152.4, 228.6) construction
  line L1 (0, 0) -> (-152.4, 0) construction
  line L2 (0, 228.6) -> (0, 0) construction
  line L3 (-152.4, 228.6) -> (0, 228.6) construction
  line L4 (-2, 2) -> (-2, 226.6) construction
  line L5 (-150.4, 2) -> (-2, 2) construction
  line L6 (-150.4, 226.6) -> (-150.4, 2) construction
  line L7 (-2, 226.6) -> (-150.4, 226.6) construction
  line L8 (0, 0) -> (-150.4, 0)
  line L9 (-71.898, 8) -> (-78.502, 8)
  line L10 (-78.502, 8) -> (-78.502, -8)
  line L11 (-78.502, -8) -> (-71.898, -8)
  line L12 (-71.898, -8) -> (-71.898, 8)
  line L13 (-71.898, 8) -> (-78.502, -8) construction
  line L14 (-78.502, 8) -> (-71.898, -8) construction
  line L15 (-75.2, 0) -> (-150.4, 0)
  line L16 (-75.2, 0) -> (0, 0)
  line L17 (-34.298, -8) -> (-40.902, -8)
  line L18 (-40.902, -8) -> (-40.902, 8)
  line L19 (-40.902, 8) -> (-34.298, 8)
  line L20 (-34.298, 8) -> (-34.298, -8)
  line L21 (-34.298, -8) -> (-40.902, 8) construction
  line L22 (-40.902, -8) -> (-34.298, 8) construction
  line L23 (-109.498, 8) -> (-116.102, 8)
  line L24 (-116.102, 8) -> (-116.102, -8)
  line L25 (-116.102, -8) -> (-109.498, -8)
  line L26 (-109.498, -8) -> (-109.498, 8)
  line L27 (-109.498, 8) -> (-116.102, -8) construction
  line L28 (-116.102, 8) -> (-109.498, -8) construction
  point P0 (-37.6, 0)
  point P1 (-112.8, 0)
  point P2 (-116.102, 0)
  point P3 (-109.498, 0)
  point P4 (-78.502, 0)
  point P5 (-71.898, 0)
  point P6 (-40.902, 0)
  point P7 (-34.298, 0)
  point P8 (-37.6, 8)
  dimension "d173" = 6.604
  dimension "d174" = 16
  dimension "d175" = 6.604
  dimension "d176" = 16
  dimension "d177" = 6.604
  dimension "d178" = 16
  constraints: 42 end point, 10 midpoint, 6 parallel, 3 horizontal, 3 perpendicular, 2 collinear, 1 point on line
  measures "d173" distance of L9.start L9.end
  measures "d174" distance of L10.end L9.end
  measures "d175" distance of L17.start L17.end
  measures "d176" distance of L17.end L18.end
  measures "d177" distance of L23.start L23.end
  measures "d178" distance of L24.end L23.end
extrude "LeftCuts" cut sketch "Sketch24" against normal blind 2 contours L8 L18 L19 L20 | L8 L24 L23 L26 | L8 L10 L9 L12
ref_plane "LRMidplane" through (-152.4, 0, -114.3) normal (0, 0, 1) x (1, 0, 0)
mirror "RightCuts" about plane through (-152.4, 0, -114.3) normal (0, 0, 1) of "LeftCuts"
sketch "Sketch25" plane through (0, 4, 0) normal (0, 1, 0) x (1, 0, 0)
  line L0 (-152.4, 0) -> (-152.4, 228.6) construction
  line L1 (0, 0) -> (-152.4, 0) construction
  line L2 (0, 228.6) -> (0, 0) construction
  line L3 (-152.4, 228.6) -> (0, 228.6) construction
  line L4 (-2, 2) -> (-2, 226.6) construction
  line L5 (-34.298, 2) -> (-2, 2) construction
  line L6 (-150.4, 226.6) -> (-150.4, 2) construction
  line L7 (-2, 226.6) -> (-34.298, 226.6) construction
  line L8 (-152.4, 0) -> (-152.4, 32.7152) construction
  line L9 (-152.4, 228.6) -> (-152.4, 0) construction
  line L10 (-152.4, 32.7152) -> (-152.4, 37.7952) construction
  line L11 (-152.4, 37.7952) -> (-152.4, 100.6602) construction
  line L12 (-152.4, 100.6602) -> (-152.4, 105.7402) construction
  line L13 (-152.4, 105.7402) -> (-152.4, 168.6052) construction
  line L14 (-152.4, 168.6052) -> (-152.4, 173.6852) construction
  line L15 (-152.4, 32.7152) -> (-144.4, 32.7152)
  line L16 (-144.4, 32.7152) -> (-144.4, 37.7952)
  line L17 (-144.4, 37.7952) -> (-152.4, 37.7952)
  line L18 (-152.4, 37.7952) -> (-152.4, 32.7152)
  line L19 (-152.4, 100.6602) -> (-144.4, 100.6602)
  line L20 (-144.4, 100.6602) -> (-144.4, 105.7402)
  line L21 (-144.4, 105.7402) -> (-152.4, 105.7402)
  line L22 (-152.4, 105.7402) -> (-152.4, 100.6602)
  line L23 (-152.4, 173.6852) -> (-144.4, 173.6852)
  line L24 (-144.4, 173.6852) -> (-144.4, 168.6052)
  line L25 (-144.4, 168.6052) -> (-152.4, 168.6052)
  line L26 (-152.4, 168.6052) -> (-152.4, 173.6852)
  line L27 (-34.298, 8) -> (-34.298, 2) projected
  line L28 (-40.902, 8) -> (-34.298, 8) projected
  line L29 (-40.902, 2) -> (-40.902, 8) projected
  line L30 (-71.898, 2) -> (-40.902, 2) projected
  line L31 (-71.898, 8) -> (-71.898, 2) projected
  line L32 (-78.502, 8) -> (-71.898, 8) projected
  line L33 (-78.502, 2) -> (-78.502, 8) projected
  line L34 (-109.498, 2) -> (-78.502, 2) projected
  line L35 (-109.498, 8) -> (-109.498, 2) projected
  line L36 (-116.102, 8) -> (-109.498, 8) projected
  line L37 (-116.102, 2) -> (-116.102, 8) projected
  line L38 (-150.4, 2) -> (-116.102, 2) projected
  line L39 (-78.502, 226.6) -> (-109.498, 226.6) projected
  line L40 (-78.502, 226.6) -> (-78.502, 220.6) projected
  line L41 (-78.502, 220.6) -> (-71.898, 220.6) projected
  line L42 (-71.898, 220.6) -> (-71.898, 226.6) projected
  line L43 (-40.902, 226.6) -> (-71.898, 226.6) projected
  line L44 (-40.902, 226.6) -> (-40.902, 220.6) projected
  line L45 (-40.902, 220.6) -> (-34.298, 220.6) projected
  line L46 (-34.298, 220.6) -> (-34.298, 226.6) projected
  line L47 (-116.102, 226.6) -> (-150.4, 226.6) projected
  line L48 (-116.102, 226.6) -> (-116.102, 220.6) projected
  line L49 (-116.102, 220.6) -> (-109.498, 220.6) projected
  line L50 (-109.498, 220.6) -> (-109.498, 226.6) projected
  dimension "d155" = 32.7152
  dimension "d156" = 5.08
  dimension "d157" = 62.865
  dimension "d158" = 5.08
  dimension "d159" = 62.865
  dimension "d160" = 5.08
  dimension "d161" = 8
  dimension "d162" = 8
  dimension "d163" = 8
  constraints: 36 end point, 6 parallel, 6 point on line, 3 horizontal, 3 perpendicular
  measures "d155" distance of L0.start L8.end
  measures "d156" distance of L8.end L10.end
  measures "d157" distance of L10.end L11.end
  measures "d158" distance of L11.end L12.end
  measures "d159" distance of L12.end L13.end
  measures "d160" distance of L13.end L14.end
  measures "d161" distance of L17.end L16.end
  measures "d162" distance of L21.end L20.end
  measures "d163" distance of L24.end L25.end
extrude "Extrusion24" cut sketch "Sketch25" against normal blind 2
body "Solid1"
